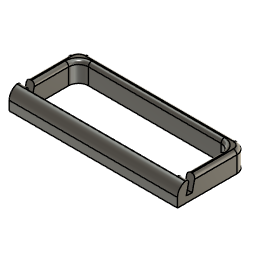
BadgeStand v6 (Autodesk Fusion 360 design; units mm, degrees)
Autodesk Fusion 360 part; units mm, degrees
note: some values were not read from the file. Chosen so that the rebuilt part matches the saved one: which face or edge a step refers to; which pieces of a blend or face edit are solid.
sketch "Sketch13" plane through (0, 0, 0) normal (0, 0, 1) x (1, 0, 0)
  line L0 (-175.2204, 23.4219) -> (-98.2204, 23.4219)
  line L1 (-98.2204, 23.4219) -> (-98.2204, -3.5781)
  line L2 (-98.2204, -3.5781) -> (-175.2204, -3.5781)
  line L3 (-175.2204, -3.5781) -> (-175.2204, 23.4219)
  line L4 (-175.2204, 23.4219) -> (-179.2204, 23.4219)
  line L5 (-179.2204, 23.4219) -> (-179.2204, -3.5781)
  line L6 (-179.2204, -3.5781) -> (-175.2204, -3.5781)
  line L7 (-175.2204, -3.5781) -> (-175.2204, 23.4219)
  line L8 (-98.2204, 23.4219) -> (-94.2204, 23.4219)
  line L9 (-94.2204, 23.4219) -> (-94.2204, -3.5781)
  line L10 (-94.2204, -3.5781) -> (-98.2204, -3.5781)
  line L11 (-98.2204, -3.5781) -> (-98.2204, 23.4219)
  line L12 (-179.2204, 23.4219) -> (-94.2204, 23.4219)
  line L13 (-94.2204, 23.4219) -> (-94.2204, 27.4219)
  line L14 (-94.2204, 27.4219) -> (-179.2204, 27.4219)
  line L15 (-179.2204, 27.4219) -> (-179.2204, 23.4219)
  line L16 (-179.2204, -3.5781) -> (-94.2204, -3.5781)
  line L17 (-94.2204, -3.5781) -> (-94.2204, -7.5781)
  line L18 (-94.2204, -7.5781) -> (-179.2204, -7.5781)
  line L19 (-179.2204, -7.5781) -> (-179.2204, -3.5781)
  dimension "d63" = 77
  dimension "d64" = 27
  dimension "d65" = 4
  dimension "d66" = 27
  dimension "d67" = 4
  dimension "d68" = 27
  dimension "d69" = 4
  dimension "d70" = 4
  constraint horizontal L0
  constraint vertical L1
  constraint horizontal L2
  constraint vertical L3
  constraint horizontal L4
  constraint vertical L5
  constraint horizontal L6
  constraint vertical L7
  constraint horizontal L8
  constraint vertical L9
  constraint horizontal L10
  constraint vertical L11
  constraint horizontal L12
  constraint vertical L13
  constraint horizontal L14
  constraint vertical L15
  constraint horizontal L16
  constraint vertical L17
  constraint horizontal L18
  constraint vertical L19
  measures "d63" distance of L0.start L0.end
  measures "d64" distance of L0.start L2.end
  measures "d65" distance of L0.start L4.end
  measures "d66" distance of L0.start L2.end
  measures "d67" distance of L0.end L8.end
  measures "d68" distance of L0.end L1.end
  measures "d69" distance of L4.end L14.end
  measures "d70" distance of L5.end L18.end
extrude "Extrude23" add sketch "Sketch13" along normal blind 10 contours L0 L4 L8 L12 L13 L14 L15 | L3 L4 L5 L6 L7 L12 L16 | L1 L8 L9 L10 L11 L12 L16 | L2 L6 L10 L16 L17 L18 L19
sketch "Sketch15" plane through (-179.2204, 0, 0) normal (-1, 0, 0) x (0, -1, 0)
  line L0 (-27.4219, 0) -> (7.5781, 0)
  line L1 (7.5781, 0) -> (7.5781, 10)
  line L2 (7.5781, 10) -> (-27.4219, 10)
  line L3 (-27.4219, 10) -> (-27.4219, 0)
  line L4 (-0.4219, 10) -> (1.1398, 3.1764)
  line L5 (3.5781, 0) -> (3.5781, 10)
  line L6 (1.1398, 3.1764) -> (3.1398, 3.1764)
  line L7 (3.1398, 3.1764) -> (1.5781, 10)
  point P0 (-0.4219, 10)
  point P1 (1.5781, 10)
  dimension "d78" = 7
  dimension "d79" = 2
  constraint coincident P0 L4.start
  constraint perpendicular L5 L6
  constraint coincident P1 L7.end
  measures "d78" distance of P0 L4.end
  measures "d79" distance of L4.end L6.end
extrude "Extrude24" cut sketch "Sketch15" against normal blind 93.518 contours L2 L4 L6 L7
fillet "Fillet7" radius 5.372 1 edges at (-136.7204, -7.5781, 10)
move_body "Move5" bodies 1 to x (1, 0, 0) y (0, 1, 0) z (0, 0, 1) at (136.8595, 0, 0)
move_body "Move6" bodies 1 to x (1, 0, 0) y (0, 1, 0) z (0, 0, 1) at (0, -9.6452, 0)
fillet "Fillet8" radius 5 2 edges at (42.6391, 17.7767, 5) (-42.3609, 17.7767, 5)
fillet "Fillet9" radius 5 2 edges at (38.6391, 13.7767, 5) (-38.3609, 13.7767, 5)
fillet "Fillet12" radius 1.338 2 edges at (-40.3609, -11.2233, 10) (40.6391, -11.2233, 10)
extrude "Extrude25" cut 2 faces at (41.3058, -9.7439, 7.7255) (-39.6942, -9.7439, 7.7255) along direction (0, 0.974797, -0.223094) blind 1.009
extrude "Extrude26" cut 1 faces at (-41.0276, -10.4571, 3.1014) along direction (0, 0.223094, 0.974797) blind 9.18
fillet "Fillet13" radius 316.698 1 edges at (-40.3609, -10.785, 3.1764)
extrude "Extrude27" cut 1 faces at (39.9724, -10.4571, 3.1014) along direction (0, 0.223094, 0.974797) blind 9.711
fillet "Fillet14" radius 569.145 1 edges at (40.6391, -10.785, 3.1764)
fillet "Fillet15" radius 1.75 10 edges at (42.6391, 2.2942, 10) (41.1746, 16.3122, 10) (0.1391, 17.7767, 10) (-40.8964, 16.3122, 10) (-42.3609, 2.2942, 10) (-38.3609, 0.2942, 10) (-36.8964, 12.3122, 10) (0.1391, 13.7767, 10) (37.1746, 12.3122, 10) (38.6391, 0.2942, 10)
